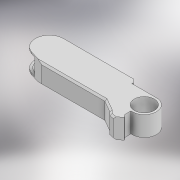
# Autodesk Inventor part: Lower Leg
Saved by Autodesk Inventor 2022 (Build 260153000, 153)
## iProperties
Created: 2022-02-26
Part Number: Lower Leg
Material: Generic
Document SubType Name: Modeling
Designer: joshw
Density: 1 g/cm^3
Appearance: Default
Author: joshw
Autodesk Inventor part; units mm, degrees
ref_plane "YZ Plane" through (0, 0, 0) normal (1, 0, 0) x (0, 1, 0)
ref_plane "XZ Plane" through (0, 0, 0) normal (0, 1, 0) x (-1, 0, 0)
ref_plane "XY Plane" through (0, 0, 0) normal (0, 0, 1) x (1, 0, 0)
sketch "Sketch1" plane through (0, 0, 0) normal (0, 1, 0) x (-1, 0, 0)
  circle A0 centre (18.7193, 0.9199) radius 3.625
  line L0 (19.1189, 4.5229) -> (19.1189, 6.4199)
  line L1 (19.1189, 6.4199) -> (18.4911, 7.1682)
  line L2 (18.4911, 7.1682) -> (20.2911, 8.6682)
  line L3 (20.2911, 8.6682) -> (21.5411, 8.4182)
  line L4 (21.5411, 8.4182) -> (22.5411, 7.4182)
  line L5 (22.5411, 7.4182) -> (26.0411, 5.4182)
  line L6 (26.0411, -4.1631) -> (26.0411, 5.4182)
  line L7 (26.0411, 5.4182) -> (45.0411, 5.4182)
  line L8 (45.0411, 5.4182) -> (49.2798, 4.1023)
  line L9 (18.8492, -2.7027) -> (26.0411, -2.7027)
  circle A1 centre (48.0263, 0.0647) radius 4.2277
  line L10 (48.0263, -4.1631) -> (26.0411, -4.1631)
  circle A2 centre (18.7193, 0.9199) radius 3
  point P0 (0, 0)
  dimension "d0" = 7.25
  dimension "d1" = 5.5
  dimension "d2" = 140
  dimension "d3" = 1.5
  dimension "d4" = 1.8
  dimension "d5" = 1.25
  dimension "d6" = 0.25
  dimension "d7" = 1
  dimension "d8" = 1
  dimension "d9" = 3.5
  dimension "d10" = 2
  dimension "d11" = 19
  dimension "d12" = 6
  dimension "d15" = 5.083
  constraints: 23 end point, 4 point on circle, 3 centre point, 2 parallel, 2 tangent, 1 coincident, 1 horizontal, 1 point on line, 1 vertical
  measures "d0" diameter of A0
  measures "d1" vertical distance of L0.end A0.centre
  measures "d2" angle of L0 L1
  measures "d3" vertical distance of L1.end L2.end
  measures "d4" horizontal distance of L1.end L2.end
  measures "d5" horizontal distance of L2.end L3.end
  measures "d6" vertical distance of L2.end L3.end
  measures "d7" horizontal distance of L3.end L4.end
  measures "d8" horizontal distance of L3.end L4.end
  measures "d9" horizontal distance of L4.end L5.end
  measures "d10" vertical distance of L4.end L5.end
  measures "d11" distance of L5.end L7.end
  measures "d12" diameter of A2
  measures "d15" distance from line of L10 A0.centre
extrude "Extrusion1" add sketch "Sketch1" along normal mid plane 5.95
ref_plane "Work Plane1" through (-52.254, 0, 0.0647) normal (1, 0, 0) x (0, 0, -1)
sketch "Sketch2" plane through (-52.254, 0, 0.0647) normal (1, 0, 0) x (0, 0, -1)
  point P0 (0.0647, 0)
sketch "Sketch3" plane through (-52.254, 0, 0.0647) normal (1, 0, 0) x (0, 0, -1)
  line L0 (-4.0376, -2.975) -> (4.2277, -2.975) construction
  line L1 (4.2277, 2.975) -> (-4.0376, 2.975) construction
  line L2 (-4.0376, -2.975) -> (-4.0376, 2.975) construction
  line L3 (2.7674, 2.975) -> (4.2277, 2.975) construction
  line L4 (-4.0376, -2.975) -> (4.2277, 2.975) construction
  line L5 (4.2277, -2.975) -> (4.2277, 2.975) construction
  line L6 (4.2277, -2.975) -> (0.095, 0) construction
  line L7 (-3.655, -2.5) -> (3.845, -2.5)
  line L8 (3.845, -2.5) -> (3.845, 2.5)
  line L9 (3.845, 2.5) -> (-3.655, 2.5)
  line L10 (-3.655, 2.5) -> (-3.655, -2.5)
  line L11 (-3.655, -2.5) -> (3.845, 2.5) construction
  line L12 (3.845, -2.5) -> (-3.655, 2.5) construction
  point P0 (0.0647, 0)
  dimension "d16" = 7.5
  dimension "d17" = 5
  constraints: 16 end point, 3 midpoint, 2 parallel, 1 horizontal, 1 perpendicular
  measures "d16" distance of L9.end L8.end
  measures "d17" distance of L8.end L7.end
extrude "Extrusion2" cut sketch "Sketch3" along normal blind 8.25
sketch "Sketch4" plane through (-50.1511, -2.5, 3.7196) normal (0, 1, 0) x (1, 0, 0)
  arc A0 (2.1248, 7.8827) -> (0.8713, -0.3827) centre (2.1248, 3.655) ccw projected
  circle A1 centre (2.1248, 3.655) radius 2.55
  point P0 (50.1511, 3.7196)
  dimension "d20" = 5.1
  constraints: 1 centre point, 1 coincident
  measures "d20" diameter of A1
extrude "Extrusion3" add sketch "Sketch4" along normal up to surface (5 mm away)
sketch "Sketch5" plane through (-49.7839, -2.5, -3.7804) normal (0, 0, 1) x (1, 0, 0)
  line L0 (0, 0) -> (0, 5) projected
  line L1 (0, 0) -> (3.5, 0)
  line L2 (3.5, 0) -> (3.5, 5)
  line L3 (0, 5) -> (3.5, 5)
  point P0 (49.7839, 2.5)
  point P1 (3.5, 0.2937)
  dimension "d23" = 3.5
  constraints: 6 end point, 1 point on line
  measures "d23" distance from line of point (3.5, 0.294) L0
extrude "Extrusion4" cut sketch "Sketch5" against normal blind 4.25
sketch "Sketch6" plane through (-44.004, 2.5, 3.7196) normal (0, 0, -1) x (-1, 0, 0)
  line L0 (6.1471, 0) -> (0, 0) projected
  line L1 (6.1471, 0) -> (4.1471, 0)
  line L2 (4.1471, 0) -> (4.1471, -5)
  line L3 (4.1471, -5) -> (6.1471, -5)
  line L4 (6.1471, -5) -> (6.1471, 0)
  line L5 (6.1471, -5) -> (0, -5) projected
  point P0 (-44.004, -2.5)
  point P1 (4.1471, 0)
  dimension "d26" = 2
  constraints: 8 end point, 2 parallel, 1 collinear, 1 horizontal, 1 perpendicular
  measures "d26" distance of L3.end L2.end
extrude "Extrusion5" cut sketch "Sketch6" against normal blind 4.25
fillet "Fillet1" radius 0.3665 2 edges at (-48.1511, 0, 4.4527) (-48.1511, 0, 3.7196)
chamfer "Chamfer1" distance 0.5 angle 45 8 edges at (-35.5411, -2.975, 5.4182) (-35.5411, 2.975, 5.4182) (-24.2911, 2.975, 6.4182) (-24.2911, -2.975, 6.4182) (-22.0411, -2.975, 7.9182) (-22.0411, 2.975, 7.9182) (-20.9161, 2.975, 8.5432) (-20.9161, -2.975, 8.5432)
chamfer "Chamfer2" distance 1 angle 45 1 edges at (-26.0411, 0, -4.1631)
fillet "Fillet2" radius 1 2 edges at (-50.5763, 2.5, 0.0647) (-50.5763, -2.5, 0.0647)
body "Solid1"
